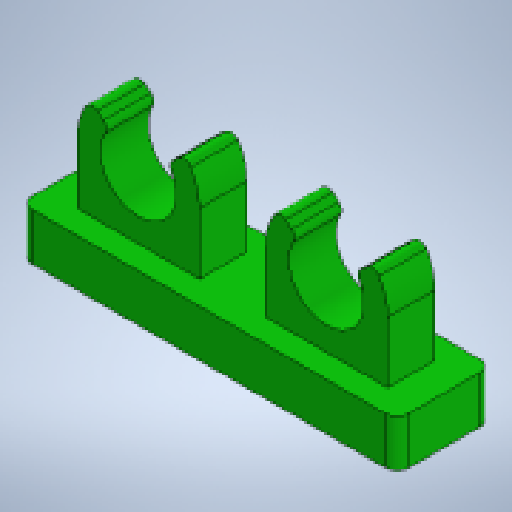
# Autodesk Inventor part: Pinecil Clip
Saved by Autodesk Inventor 2026 (Build 300175050, 175E)
## iProperties
Created: 2025-10-09
Part Number: Pinecil Clip
Material: Generic
Document SubType Name: Modeling
Designer: Nicholas M
Density: 1 g/cm^3
Appearance: Smooth - Black
Author: Nicholas M
Autodesk Inventor part; units mm, degrees
ref_plane "YZ Plane" through (0, 0, 0) normal (1, 0, 0) x (0, 1, 0)
ref_plane "XZ Plane" through (0, 0, 0) normal (0, 1, 0) x (-1, 0, 0)
ref_plane "XY Plane" through (0, 0, 0) normal (0, 0, 1) x (1, 0, 0)
sketch "Sketch1" plane through (0, 0, 0) normal (0, 0, 1) x (1, 0, 0)
  circle A0 centre (0, 0) radius 2.54
  circle A1 centre (0, 0) radius 4.1275
  line L0 (-4.1275, 0) -> (-4.1275, -4.1275)
  line L1 (-4.1275, -4.1275) -> (-6.35, -4.1275)
  line L2 (-6.35, -4.1275) -> (-6.35, -7.3025)
  line L3 (-6.35, -7.3025) -> (6.35, -7.3025)
  line L4 (6.35, -7.3025) -> (6.35, -4.1275)
  line L5 (6.35, -4.1275) -> (4.1275, -4.1275)
  line L6 (4.1275, -4.1275) -> (4.1275, 0)
  line L7 (0, 0) -> (-3.1988, 2.6084)
  line L8 (0, 0) -> (3.1988, 2.6084)
  line L9 (-4.1275, -4.1275) -> (4.1275, -4.1275)
  circle A2 centre (12.7, 0) radius 4.1275
  circle A3 centre (12.7, 0) radius 2.54
  line L10 (12.7, 0) -> (9.5012, 2.6084)
  line L11 (12.7, 0) -> (15.8988, 2.6084)
  line L12 (8.5725, -4.1275) -> (16.8275, -4.1275)
  line L13 (16.8275, -4.1275) -> (16.8275, 0)
  line L14 (8.5725, 0) -> (8.5725, -4.1275)
  line L15 (8.5725, -4.1275) -> (6.35, -4.1275)
  line L16 (6.35, -4.1275) -> (6.35, -7.3025)
  line L17 (6.35, -7.3025) -> (19.05, -7.3025)
  line L18 (19.05, -7.3025) -> (19.05, -4.1275)
  line L19 (19.05, -4.1275) -> (16.8275, -4.1275)
  point P0 (-1.9685, 1.6052)
  point P1 (1.9685, 1.6052)
  point P2 (10.7315, 1.6052)
  point P3 (14.6685, 1.6052)
  dimension "d0" = 5.08
  dimension "d1" = 1.5875
  dimension "d2" = 3.937
  dimension "d3" = 3.175
  dimension "d4" = 12.7
  dimension "d13" = 12.7
  constraints: 40 end point, 12 point on circle, 8 point on line, 5 perpendicular, 4 centre point, 3 tangent, 2 collinear, 2 horizontal, 2 horizontal alignment, 1 coincident, 1 vertical, 24 other
  measures "d0" diameter of A0
  measures "d1" radial gap between concentric circles of A0 A1
  measures "d2" distance of A0.start A0.end
  measures "d3" distance of L1.end L2.end
  measures "d4" distance of L2.end L3.end
  measures "d13" distance of L7.start L10.start
extrude "Extrusion1" add sketch "Sketch1" along normal mid plane 6.35 contours L9 L5 L4 L3 L2 L1 | L15 L12 L19 L18 L17 L4
extrude "Extrusion2" add sketch "Sketch1" along normal mid plane 3.175 contours A0 L8 A1 L7 | L6 L9 A1 | A1 L9 L0 | L14 A2 L12 | A2 L10 A3 L11 | A2 L13 L12 picked at (3.4002, 1.1083) picked at (16.2627, 0.311)
fillet "Fillet1" radius 0.7937 4 edges at (-6.35, -5.715, 3.175) (-6.35, -5.715, -3.175) (19.05, -5.715, 3.175) (19.05, -5.715, -3.175)
fillet "Fillet2" radius 0.5292 8 edges at (-1.9685, 1.6052, 0) (-3.1988, 2.6084, 0) (1.9685, 1.6052, 0) (3.1988, 2.6084, 0) (9.5012, 2.6084, 0) (10.7315, 1.6052, 0) (14.6685, 1.6052, 0) (15.8988, 2.6084, 0)
body "Solid1"
